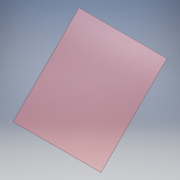
# Autodesk Inventor part: TopV2
Saved by Autodesk Inventor 2019 (Build 230136000, 136)
## iProperties
Created: 2021-09-16
Part Number: TopV2
Material: Acrylic, Clear
Document SubType Name: Modeling
Designer: timmy
Density: 1.19 g/cm^3
Appearance: Transparent - Clear
Author: timmy
Autodesk Inventor part; units mm, degrees
ref_plane "YZ Plane" through (0, 0, 0) normal (1, 0, 0) x (0, 1, 0)
ref_plane "XZ Plane" through (0, 0, 0) normal (0, 1, 0) x (-1, 0, 0)
ref_plane "XY Plane" through (0, 0, 0) normal (0, 0, 1) x (1, 0, 0)
sketch "Sketch6" plane through (0, 0, 0) normal (0, 1, 0) x (-1, 0, 0)
  line L0 (0, 0) -> (609.6, 0)
  line L1 (609.6, 0) -> (609.6, -914.4)
  line L2 (609.6, -914.4) -> (0, -914.4)
  line L3 (0, -914.4) -> (0, 0)
  dimension "d21" = 609.6
  dimension "d22" = 914.4
  constraints: 8 end point, 2 parallel, 1 horizontal, 1 perpendicular
  measures "d21" distance of L1.end L2.end
  measures "d22" distance of L0.end L1.end
extrude "Extrusion6" add sketch "Sketch6" along normal blind 609.6
sketch "Sketch8" plane through (0, 0, 0) normal (1, 0, 0) x (0, 0, -1)
  line L0 (0, 609.6) -> (914.4, 609.6) projected
  line L1 (0, 0) -> (457.2, 0) construction
  line L2 (0, 0) -> (457.2, 457.2)
  line L3 (0, 0) -> (646.5784, 0) construction
  line L4 (457.2, 457.2) -> (914.4, 0)
  line L5 (457.2, 457.2) -> (459.4451, 454.9549)
  line L6 (0, 0) -> (3.175, 0)
  line L7 (3.175, 0) -> (459.4451, 454.9549)
  dimension "d29" = 45
  dimension "d30" = 3.175
  dimension "d31" = 3.175
  constraints: 14 end point, 2 horizontal, 2 point on line, 1 equal length, 1 perpendicular
  measures "d29" angle of L3 L2
  measures "d30" distance of L2.end L5.end
  measures "d31" distance of L1.start L6.end
extrude "Extrusion7" cut sketch "Sketch8" against normal blind 609.6 keep common part
body "Solid4"
